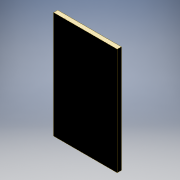
# Autodesk Inventor part: Monitor, back bump not measured
Saved by Autodesk Inventor 2017 (Build 210142000, 142)
## iProperties
Created: 2017-06-02
Part Number: Monitor, back bump not measured
Material: Generic
Document SubType Name: Modeling
Designer: crush
Density: 1 g/cm^3
Appearance: Default
Author: crush
Autodesk Inventor part; units mm, degrees
ref_plane "YZ Plane" through (0, 0, 0) normal (1, 0, 0) x (0, 1, 0)
ref_plane "XZ Plane" through (0, 0, 0) normal (0, 1, 0) x (-1, 0, 0)
ref_plane "XY Plane" through (0, 0, 0) normal (0, 0, 1) x (1, 0, 0)
sketch "Sketch1" plane through (0, 0, 0) normal (0, 1, 0) x (-1, 0, 0)
  line L0 (0, 0) -> (-380, 0)
  line L1 (-380, 0) -> (-380, -640)
  line L2 (-380, -640) -> (0, -640)
  line L3 (0, -640) -> (0, 0)
  dimension "d0" = 380
  dimension "d1" = 640
  constraints: 8 end point, 2 parallel, 1 horizontal, 1 perpendicular
  measures "d0" distance of L2.end L1.end
  measures "d1" distance of L1.end L0.end
extrude "Extrusion1" add sketch "Sketch1" along normal blind 25
sketch "Sketch2" plane through (0, 25, 0) normal (0, 1, 0) x (1, 0, 0)
  line L0 (85, 120) -> (295, 120)
  line L1 (295, 120) -> (295, 520)
  line L2 (295, 520) -> (85, 520)
  line L3 (85, 520) -> (85, 120)
  line L4 (0, 640) -> (0, 0) projected
  line L5 (380, 640) -> (0, 640) projected
  dimension "d4" = 210
  dimension "d5" = 400
  dimension "d6" = 85
  dimension "d7" = 120
  constraints: 8 end point, 2 parallel, 1 horizontal, 1 perpendicular
  measures "d4" distance of L2.end L1.end
  measures "d5" distance of L1.end L0.end
  measures "d6" distance between parallel lines of L4 L3
  measures "d7" distance between parallel lines of L5 L2
extrude "Extrusion2" add sketch "Sketch2" along normal blind 30
body "Solid1"
